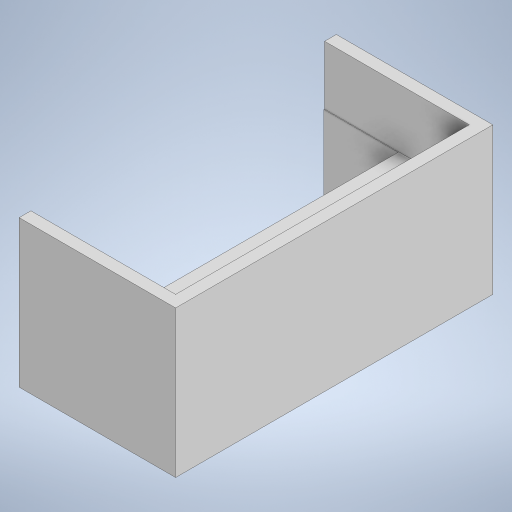
# Autodesk Inventor part: Base2
Saved by Autodesk Inventor 2023 (Build 270158000, 158)
## iProperties
Created: 2022-05-16
Part Number: Base2
Material: Generic
Document SubType Name: Modeling
Designer: WMGWW
Density: 1 g/cm^3
Appearance: Default
Author: WMGWW
Autodesk Inventor part; units mm, degrees
ref_plane "YZ Plane" through (0, 0, 0) normal (1, 0, 0) x (0, 1, 0)
ref_plane "XZ Plane" through (0, 0, 0) normal (0, 1, 0) x (-1, 0, 0)
ref_plane "XY Plane" through (0, 0, 0) normal (0, 0, 1) x (1, 0, 0)
sketch "Sketch1" plane through (0, 0, 0) normal (0, 1, 0) x (-1, 0, 0)
  line L0 (0, 0) -> (25.4, 0)
  line L1 (25.4, 0) -> (25.4, -127)
  line L2 (25.4, -127) -> (0, -127)
  line L3 (0, -127) -> (0, 0)
  line L4 (30.48, 5.08) -> (-5.08, 5.08)
  line L5 (-5.08, 5.08) -> (-5.08, -132.08)
  line L6 (-5.08, -132.08) -> (30.48, -132.08)
  line L7 (30.48, -132.08) -> (30.48, 5.08)
  dimension "d0" = 25.4
  dimension "d1" = 127
  dimension "d2" = 5.08
  dimension "d3" = 5.08
  dimension "d4" = 5.08
  dimension "d5" = 5.08
  constraints: 16 end point, 4 parallel, 2 horizontal, 2 perpendicular
  measures "d0" distance of L0.start L0.end
  measures "d1" distance of L0.end L1.end
  measures "d2" distance between parallel lines of L4 L0
  measures "d3" distance between parallel lines of L6 L2
  measures "d4" distance between parallel lines of L3 L5
  measures "d5" distance between parallel lines of L7 L1
extrude "Extrusion1" add sketch "Sketch1" along normal blind 38.1
sketch "Sketch2" plane through (0, 38.1, 0) normal (0, 1, 0) x (1, 0, 0)
  line L0 (-30.48, -5.08) -> (5.08, -5.08) projected
  line L1 (5.08, -5.08) -> (-62.5812, -5.08)
  line L2 (-62.5812, -5.08) -> (-62.5812, 0)
  line L3 (-62.5812, 0) -> (0, 0)
  line L4 (-25.4, 127) -> (0, 127) projected
  line L5 (0, 127) -> (-62.5812, 127)
  line L6 (5.08, -5.08) -> (5.08, 132.08) projected
  line L7 (5.08, -5.08) -> (-62.5812, -5.08)
  line L8 (-62.5812, 132.08) -> (5.08, 132.08)
  line L9 (5.08, 132.08) -> (5.08, -5.08)
  line L10 (-62.5812, 132.08) -> (-47.0844, 132.08)
  line L11 (-62.5812, 127) -> (-62.5812, 132.08)
  line L12 (0, 127) -> (0, 0) projected
  line L13 (0, 0) -> (0, 127)
  line L14 (0, 127) -> (-62.5812, 127)
  line L15 (-62.5812, 132.08) -> (3.2473, 132.08)
  line L16 (5.08, 132.08) -> (-30.48, 132.08) projected
  constraints: 24 end point, 3 horizontal, 2 perpendicular, 2 point on line, 1 collinear, 1 parallel
extrude "Extrusion2" add sketch "Sketch2" along normal blind 25.4
sketch "Sketch5" plane through (0, 38.1, 0) normal (0, -1, 0) x (1, 0, 0)
  line L0 (-62.5812, -132.08) -> (-62.5812, -127) projected
  line L1 (-30.48, -132.08) -> (-30.48, 5.08) projected
  line L2 (-62.5812, -132.08) -> (-30.48, -132.08)
  line L3 (-30.48, -132.08) -> (-30.48, -126.7104)
  line L4 (-30.48, -126.7104) -> (-62.5812, -126.7104)
  line L5 (-62.5812, -126.7104) -> (-62.5812, -132.08)
  line L6 (-62.5812, 0) -> (-62.5812, 5.08) projected
  line L7 (-30.48, 5.08) -> (5.08, 5.08) projected
  line L8 (-62.5812, 0) -> (-30.48, 0)
  line L9 (-30.48, 0) -> (-30.48, 5.08)
  line L10 (-30.48, 5.08) -> (-62.5812, 5.08)
  line L11 (-62.5812, 5.08) -> (-62.5812, 0)
  point P0 (0, 0)
  constraints: 16 end point, 4 parallel, 2 horizontal, 2 perpendicular, 1 point on line
extrude "Extrusion3" add sketch "Sketch5" along normal blind 38.1
body "Solid1"
